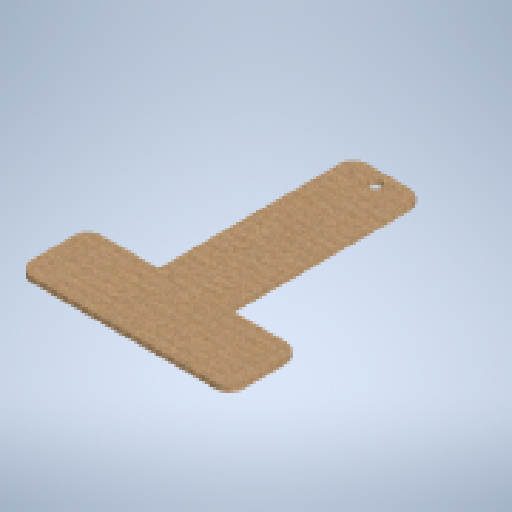
# Autodesk Inventor part: PistonBC
Saved by Autodesk Inventor 2023.1 (Build 271208000, 208)
## iProperties
Created: 2022-11-11
Part Number: PistonBC
Material: MDF Medium Density Fiberboard
Document SubType Name: Modeling
Designer: Daniel Peña
Density: 0.8 g/cm^3
Appearance: Cardboard - Corrugated
Author: Daniel Peña
Autodesk Inventor part; units mm, degrees
ref_plane "YZ Plane" through (0, 0, 0) normal (1, 0, 0) x (0, 1, 0)
ref_plane "XZ Plane" through (0, 0, 0) normal (0, 1, 0) x (-1, 0, 0)
ref_plane "XY Plane" through (0, 0, 0) normal (0, 0, 1) x (1, 0, 0)
sketch "Sketch1" plane through (0, 0, 0) normal (0, 0, 1) x (1, 0, 0)
  line L0 (8, 60) -> (32, 60)
  line L1 (32, -60) -> (8, -60)
  line L2 (0, -52) -> (0, 52)
  line L3 (40, 20) -> (142, 20)
  line L4 (150, 12) -> (150, -12)
  line L5 (142, -20) -> (40, -20)
  line L6 (40, 52) -> (40, 20)
  line L7 (40, -20) -> (40, -52)
  line L8 (0, 0) -> (150, 0) construction
  arc A0 (8, 60) -> (0, 52) centre (8, 52) ccw
  arc A1 (0, -52) -> (8, -60) centre (8, -52) ccw
  arc A2 (40, 52) -> (32, 60) centre (32, 52) ccw
  arc A3 (142, -20) -> (150, -12) centre (142, -12) ccw
  arc A4 (150, 12) -> (142, 20) centre (142, 12) ccw
  arc A5 (32, -60) -> (40, -52) centre (32, -52) ccw
  point P0 (0, 0)
  point P1 (40, -60)
  point P2 (0, -60)
  point P3 (150, -20)
  point P4 (150, 20)
  dimension "d0" = 40
  dimension "d1" = 40
  dimension "d2" = 150
  dimension "d3" = 8
  dimension "d4" = 8
  dimension "d5" = 120
  constraints: 18 end point, 12 point on circle, 12 tangent, 8 point on line, 6 centre point, 4 equal radius, 4 parallel, 3 horizontal, 3 perpendicular, 2 midpoint, 1 collinear, 1 other
  measures "d0" distance of point (150, 20) point (150, -20)
  measures "d1" distance of point (40, -60) point (0, -60)
  measures "d2" distance between parallel lines of L4 L2
  measures "d3" radius of A0
  measures "d4" radius of A5
  measures "d5" distance between parallel lines of L1 L0
extrude "Extrusion1" add sketch "Sketch1" along normal blind 3
sketch "Sketch2" plane through (0, 0, 3) normal (0, 0, 1) x (1, 0, 0)
  line L0 (150, -12) -> (150, 12) projected
  line L1 (40, -20) -> (142, -20) projected
  point P0 (0, 0)
  point P1 (142.5, 0)
  dimension "d8" = 7.5
  dimension "d9" = 20
  measures "d8" distance from line of L0 point (142.5, 0)
  measures "d9" distance from line of point (142.5, 0) L1
hole "Hole1" at (142.5, 0, 3) direction (0, 0, -1) diameter 7 end through all
body "Solid1"
